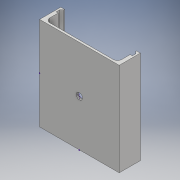
# Autodesk Inventor part: HB5_holder
Saved by Autodesk Inventor 2018 (Build 220112000, 112)
## iProperties
Created: 2018-04-27
Part Number: HB5_holder
Material: 一般
Document SubType Name: Modeling
Designer: izumi
Density: 1 g/cm^3
Appearance: 既定
Author: izumi
Autodesk Inventor part; units mm, degrees
ref_plane "YZ Plane" through (0, 0, 0) normal (1, 0, 0) x (0, 1, 0)
ref_plane "XZ Plane" through (0, 0, 0) normal (0, 1, 0) x (-1, 0, 0)
ref_plane "XY Plane" through (0, 0, 0) normal (0, 0, 1) x (1, 0, 0)
sketch "本体面" plane through (0, 0, 0) normal (0, 0, 1) x (1, 0, 0)
  line L0 (-18.8, 10) -> (18.8, 10)
  line L1 (18.8, 10) -> (18.8, 0)
  line L2 (18.8, 0) -> (-18.8, 0)
  line L3 (-18.8, 0) -> (-18.8, 10)
  point P0 (0, 0)
  point P1 (0, 0)
  dimension "d0" = 37.6
  dimension "d1" = 10
  constraints: 8 end point, 2 parallel, 1 coincident, 1 horizontal, 1 midpoint, 1 perpendicular
  measures "d0" distance of L1.end L2.end
  measures "d1" distance of L0.end L1.end
extrude "本体" add sketch "本体面" along normal blind 44
sketch "空洞面" plane through (0, 0, 44) normal (0, 0, 1) x (1, 0, 0)
  line L0 (-17, 10) -> (17, 10)
  line L1 (17, 10) -> (17, 3)
  line L2 (15, 1) -> (-15, 1)
  line L3 (-17, 3) -> (-17, 10)
  line L4 (18.8, 10) -> (-18.8, 10) projected
  arc A0 (-17, 3) -> (-15, 1) centre (-15, 3) ccw
  arc A1 (15, 1) -> (17, 3) centre (15, 3) ccw
  point P0 (0, 0)
  point P1 (17, 1)
  point P2 (-17, 1)
  point P3 (0, 10)
  dimension "d4" = 34
  dimension "d5" = 9
  dimension "d6" = 2
  constraints: 8 end point, 4 point on circle, 4 point on line, 4 tangent, 2 centre point, 2 midpoint, 2 parallel, 1 equal radius, 1 horizontal, 1 perpendicular
  measures "d4" distance of point (17, 1) point (-17, 1)
  measures "d5" distance of L0.end point (17, 1)
  measures "d6" radius of A0
extrude "空洞" cut sketch "空洞面" against normal up to surface (44 mm away)
sketch "溝形状" plane through (0, 0, 44) normal (0, 0, 1) x (1, 0, 0)
  line L0 (-17, 10) -> (-18.8, 10) construction
  line L1 (-18.8, 10) -> (-18.8, 0) construction
  line L2 (-17, 3) -> (-17, 10) construction
  line L3 (17, 9.6) -> (-17, 9.6)
  line L4 (-17, 9.6) -> (-18, 8.6)
  line L5 (18, 8.6) -> (17, 9.6)
  line L6 (18.8, 0) -> (18.8, 10) construction
  line L7 (18.8, 10) -> (17, 10) construction
  line L8 (17, 10) -> (17, 3) construction
  line L9 (-18, 8.6) -> (-18, 7)
  line L10 (-18, 7) -> (18, 7)
  line L11 (18, 7) -> (18, 8.6)
  line L12 (-10, 9) -> (10, 9) construction
  line L13 (10, 9) -> (10, 7) construction
  line L14 (10, 7) -> (-10, 7) construction
  line L15 (-10, 7) -> (-10, 9) construction
  point P0 (0, 0)
  point P1 (0, 7)
  dimension "d31" = 135
  dimension "d34" = 0.8
  dimension "d35" = 0.4
  dimension "d36" = 0.8
  dimension "d37" = 135
  dimension "d38" = 2.6
  dimension "d41" = 2
  dimension "d42" = 20
  constraints: 20 end point, 3 horizontal, 2 midpoint, 2 parallel, 2 perpendicular, 1 horizontal alignment, 1 point on line, 1 vertical
  measures "d31" angle of L3 L4
  measures "d34" distance from line of L6 L5.start
  measures "d35" distance between parallel lines of L7 L3
  measures "d36" distance from line of L1 L4.end
  measures "d37" angle of L3 L5
  measures "d38" distance between parallel lines of L10 L3
  measures "d41" distance between parallel lines of L14 L12
  measures "d42" distance between parallel lines of L15 L13
extrude "溝" cut sketch "溝形状" against normal blind 43
sketch "底中央" plane through (-18.8, 0, 0) normal (0, -1, 0) x (1, 0, 0)
  line L0 (0, 0) -> (0, 44) construction
  line L1 (37.6, 0) -> (0, 0) construction
  point P0 (18.8, 0)
  point P1 (18.8, 22)
  point P2 (0, 22)
  point P3 (18.8, 0)
  constraints: 2 midpoint, 1 horizontal alignment, 1 vertical alignment
sketch "スケッチ8" plane through (-15, 1, 44) normal (0, 1, 0) x (1, 0, 0)
  line L0 (30, 0) -> (30, 44) projected
  line L1 (-2, 44) -> (0, 44) projected
  line L2 (0, 0) -> (0, 44) projected
  line L3 (30, 44) -> (32, 44) projected
  circle A0 centre (15, 22) radius 1.5
  point P0 (15, 44)
  dimension "d50" = 3
  constraints: 1 centre point
  measures "d50" diameter of A0
extrude "押し出し5" cut sketch "スケッチ8" against normal through all
